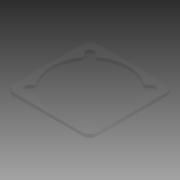
# Autodesk Inventor part: D-057
Saved by Autodesk Inventor 2015 (Build 190159000, 159)
## iProperties
Company: MARCHA TECHNOLOGY
Created: 2013-10-15
Part Number: D-057
Document SubType Name: Modeling
Designer: O.Martin
Density: 1 g/cm^3
Mass: 0.789088 g
Surface Area: 14.5064 cm^2
Volume: 0.789088 cm^3
Project: WITBOXprinter_K01
Description: SUPLEMENTO FAN50
Stock Number: 28655
Material: Generic
Appearance: Clear - Light
Author: O.Martin
Autodesk Inventor part; units mm, degrees
ref_plane "YZ Plane" through (0, 0, 0) normal (1, 0, 0) x (0, 1, 0)
ref_plane "XZ Plane" through (0, 0, 0) normal (0, 1, 0) x (-1, 0, 0)
ref_plane "XY Plane" through (0, 0, 0) normal (0, 0, 1) x (1, 0, 0)
sketch "Boceto1" plane through (0, 0, 0) normal (0, 0, 1) x (1, 0, 0)
  line L0 (-27.5, 27.5) -> (27.5, 27.5)
  line L1 (27.5, 27.5) -> (27.5, -27.5)
  line L2 (27.5, -27.5) -> (-27.5, -27.5)
  line L3 (-27.5, -27.5) -> (-27.5, 27.5)
  circle A0 centre (0, 0) radius 25
  line L4 (-20, 20) -> (20, 20) construction
  line L5 (20, 20) -> (20, -20) construction
  line L6 (20, -20) -> (-20, -20) construction
  line L7 (-20, -20) -> (-20, 20) construction
  circle A1 centre (-20, 20) radius 2.625
  circle A2 centre (20, 20) radius 2.625
  circle A3 centre (20, -20) radius 2.625
  circle A4 centre (-20, -20) radius 2.625
  line L8 (-18.1438, 21.8562) -> (-15.7238, 19.4361)
  line L9 (-21.8562, 18.1438) -> (-19.4361, 15.7238)
  line L10 (21.8562, -18.1438) -> (19.4361, -15.7238)
  line L11 (18.1438, -21.8562) -> (15.7238, -19.4361)
  line L12 (18.1438, 21.8562) -> (15.7238, 19.4361)
  line L13 (21.8562, 18.1438) -> (19.4361, 15.7238)
  line L14 (-21.8562, -18.1438) -> (-19.4361, -15.7238)
  line L15 (-18.1438, -21.8562) -> (-15.7238, -19.4361)
  point P0 (0, 27.5)
  point P1 (27.5, 0)
  point P2 (0, 20)
  point P3 (20, 0)
  dimension "d0" = 50
  dimension "d1" = 55
  dimension "d2" = 40
  dimension "d3" = 5.25
  dimension "d7" = 45
  constraints: 32 end point, 10 parallel, 8 point on circle, 7 tangent, 5 coincident, 4 centre point, 4 midpoint, 3 equal length, 3 equal radius, 3 perpendicular, 2 horizontal, 2 horizontal alignment, 2 vertical alignment, 10 other
  measures "d1" distance of L0.start L0.end
  measures "d2" distance of L4.start L4.end
  measures "d3" diameter of A1
  measures "d7" angle of L0 L8
extrude "Extrusión1" add sketch "Boceto1" along normal blind 2
fillet "Empalme1" radius 5 4 edges at (-27.5, 27.5, 1) (-27.5, -27.5, 1) (27.5, -27.5, 1) (27.5, 27.5, 1)
fillet "Empalme1" radius 2 8 edges at (-19.4361, 15.7238, 1) (-15.7238, 19.4361, 1) (15.7238, 19.4361, 1) (19.4361, 15.7238, 1) (19.4361, -15.7238, 1) (15.7238, -19.4361, 1) (-15.7238, -19.4361, 1) (-19.4361, -15.7238, 1)
body "Solid1"
